Autodesk Fusion 360 part; units mm, degrees
(part 2 of 2)
  constraint symmetric L8 A252 A259
  constraint symmetric L8 L179.end A261.start
  constraint symmetric L8 L180.start L183.start
  constraint symmetric L8 A253 A261
  constraint symmetric L8 L177.end L184.end
  constraint symmetric L8 L178.start L182.start
  constraint symmetric L8 A254 A263
  constraint symmetric L8 L178.end L182.end
  constraint symmetric L8 L179.start L185.start
  constraint symmetric L8 A255 A262
  constraint symmetric L8 A256 A260
  constraint symmetric L8 A257 A258
  constraint symmetric L8 A264 A265
  constraint symmetric L7 A264 A267
  constraint symmetric L7 A265 A266
  measures "d1" diameter of A0
  measures "d2" distance of L0.start L0.end
  measures "d3" distance of L0.start L2.end
  measures "d4" diameter of A1
  measures "d5" diameter of A2
  measures "d6" diameter of A3
  measures "d7" distance of L1 A3.centre
  measures "d8" distance of L3 A2.centre
  measures "d9" distance of A0.centre L0
  measures "d10" distance of L2 A2.centre
  measures "d11" distance of L1 L4
  measures "d12" diameter of A4
  measures "d13" distance of A4.centre L6
  measures "d15" distance of L9.start L11.end L6.end
  measures "d16" distance of L1 L18
  measures "d17" distance of L15 L17
  measures "d18" distance of L19.start L19.end
  measures "d19" distance of L23.end L24.end
  measures "d20" distance of L23.start L23.end
  measures "d21" distance of L19 L21
  measures "d22" diameter of A5
  measures "d26" distance of L12 L26
  measures "d27" distance of L9 L27
  measures "d28" distance of L10 L12
  measures "d29" distance of L26 L41
  measures "d30" distance of L23 L40
  measures "d31" radius of A6
  measures "d32" radius of A8
  measures "d33" radius of A10
  measures "d34" distance of L68 L71
  measures "d35" radius of A33
  measures "d36" distance of A36.centre A35.centre
  measures "d37" radius of A35
  measures "d40" diameter of A47
  measures "d41" diameter of A48
  measures "d42" diameter of A49
  measures "d43" diameter of A50
  measures "d44" diameter of A51
  measures "d45" distance of A52.centre A51.centre
  measures "d46" distance of L73 A52.centre
  measures "d47" distance of L71 L81
  measures "d48" diameter of A53
  measures "d49" distance of L68 L84
  measures "d50" diameter of A59
  measures "d51" distance of L8 A59.centre
  measures "d56" distance of L68 A59.centre
  measures "d57" diameter of A60
  measures "d58" vertical distance of A59.centre A60.centre
  measures "d59" distance of L8 A60.centre
  measures "d60" diameter of A63
  measures "d61" diameter of A64
  measures "d62" angle of L89 L90
  measures "d63" distance of L7 A63.centre
  measures "d64" distance of L7 A64.centre
  measures "d65" diameter of A71
  measures "d66" diameter of A72
  measures "d67" distance of A73.centre A72.centre
  measures "d68" distance of L12 L93
  measures "d70" diameter of A74
  measures "d72" diameter of A75
  measures "d73" vertical distance of A73.centre A75.centre
  measures "d74" distance of A72.centre A74.centre
  measures "d75" diameter of A86
  measures "d76" distance of A87.centre A86.centre
  measures "d77" distance of L12 L102
  measures "d78" distance of L40 A86.centre
  measures "d79" diameter of A90
  measures "d80" distance of L45 L107
  measures "d81" distance of A91.centre A90.centre
  measures "d82" diameter of A92
  measures "d83" distance of A90.centre A92.centre L6.end
  measures "d84" diameter of A93
  measures "d85" distance of A94.centre A93.centre
  measures "d86" distance of A92.centre A94.centre
  measures "d87" diameter of A95
  measures "d88" distance of A93.centre A95.centre
  measures "d89" diameter of A96
  measures "d90" distance of A95.centre A97.centre
  measures "d91" distance of A97.centre A96.centre
  measures "d92" diameter of A98
  measures "d93" distance of A96.centre A98.centre
  measures "d94" diameter of A106
  measures "d95" distance of L53 A106.centre
  measures "d100" diameter of A107
  measures "d101" distance of L68 A107.centre
  measures "d102" diameter of A108
  measures "d103" diameter of A109
  measures "d104" distance of A108.centre A109.centre
  measures "d105" vertical distance of A5.centre A109.centre
  measures "d106" diameter of A111
  measures "d107" diameter of A110
  measures "d108" distance of A110.centre A111.centre
  measures "d109" vertical distance of A107.centre A111.centre
  measures "d110" diameter of A118
  measures "d111" diameter of A117
  measures "d112" distance of A118.centre A117.centre
  measures "d113" vertical distance of A31.centre A118.centre
  measures "d114" diameter of A121
  measures "d116" distance of L8 A121.centre
  measures "d117" vertical distance of A36.centre A121.centre
  measures "d118" diameter of A123
  measures "d119" diameter of A124
  measures "d120" angle of L119 L120
  measures "d121" diameter of A125
  measures "d122" diameter of A126
  measures "d123" diameter of A127
  measures "d124" diameter of A128
  measures "d127" distance of L45 A123.centre
  measures "d128" distance of P1 P2
  measures "d129" distance of P1 P3
  measures "d130" radius of A134
  measures "d131" diameter of A138
  measures "d132" distance of L121 A138.centre
  measures "d133" distance of L124 A138.centre
  measures "d134" diameter of A140
  measures "d135" distance of L121 A140.centre
  measures "d136" distance of A138.centre A140.centre
  measures "d137" angle of L127 L128
  measures "d138" distance of L127.start L127.end
  measures "d139" diameter of A154
  measures "d140" diameter of A155
  measures "d141" distance of A154.centre A155.centre
  measures "d142" distance of L121 A155.centre
  measures "d143" diameter of A156 L6.end
  measures "d144" diameter of A157
  measures "d145" distance of A156.centre A157.centre
  measures "d146" distance of L7 A157.centre
  measures "d149" diameter of A184
  measures "d150" distance of L9 A184.centre
  measures "d151" distance of L8 A184.centre
  measures "d152" diameter of A186
  measures "d153" distance of L72 A186.centre
  measures "d154" distance of L71 A186.centre
  measures "d155" diameter of A188
  measures "d156" distance of L47 A188.centre
  measures "d157" distance of L10 A188.centre
  measures "d158" diameter of A190
  measures "d159" distance of L66 A190.centre
  measures "d160" distance of L12 A190.centre
  measures "d163" diameter of A191
  measures "d164" distance of L42 A191.centre
  measures "d165" diameter of A201
  measures "d166" distance of L68 A201.centre
  measures "d169" distance of L143.start L143.end
  measures "d170" distance of L143.start L145.end
  measures "d171" diameter of A207
  measures "d172" distance of L147.start L147.end
  measures "d173" distance of L12 L144
  measures "d176" diameter of A216
  measures "d177" vertical distance of A157.centre P8
  measures "d179" diameter of A217
  measures "d180" angle of L157 L158
  measures "d181" diameter of A218
  measures "d182" angle of L159 L160
  measures "d183" diameter of A222
  measures "d184" radius of A227
  measures "d186" distance of A226.end L162.end
  measures "d187" distance of L7 L163
  measures "d188" diameter of A228
  measures "d189" distance of L12 A228.centre
  measures "d190" distance of L61 A228.centre
  measures "d191" diameter of A229
  measures "d192" distance of L12 A229.centre
  measures "d193" diameter of A230
  measures "d194" distance of A229.centre A230.centre
  measures "d195" diameter of A231
  measures "d196" distance of A228.centre A231.centre
  measures "d197" diameter of A232
  measures "d198" distance of A231.centre A232.centre
  measures "d199" diameter of A233
  measures "d200" distance of A231.centre A233.centre
  measures "d201" diameter of A234
  measures "d202" distance of A232.centre A234.centre
  measures "d203" diameter of A235
  measures "d204" diameter of A236
  measures "d205" diameter of A237
  measures "d206" distance of A232.centre A235.centre
  measures "d207" distance of A235.centre A237.centre
  measures "d208" diameter of A238
  measures "d209" distance of L164.start L164.end
  measures "d212" diameter of A242
  measures "d213" diameter of A243
  measures "d214" distance of A242.centre A243.centre
  measures "d215" distance of L8 A242.centre
  measures "d216" distance of L7 A242.centre
  measures "d221" diameter of A246
  measures "d222" distance of A246.end L170.end
  measures "d223" diameter of A248
  measures "d224" distance of L172.start L172.end
  measures "d225" distance of P10 P11
  measures "d226" distance of P10 P12
  measures "d227" radius of A252
  measures "d228" diameter of A256
  measures "d229" diameter of A257
  measures "d230" horizontal distance of A256.centre A257.centre
  measures "d231" diameter of A264
extrude "拉伸9" add sketch "草图1" along normal blind 3
sketch "草图5" plane through (0, 0, 3) normal (0, 0, 1) x (-1, 0, 0)
  circle A0 centre (-65.0738, -123.4519) radius 11
  circle A1 centre (-71.75, -44.17) radius 1.3
  circle A2 centre (24.5, 82.5) radius 1.6
  circle A3 centre (-112.5, 146) radius 1.6
  circle A4 centre (86, 58.5) radius 2.1
  circle A5 centre (-30.5, -30.5) radius 2.1
  circle A6 centre (-92.25, -44.17) radius 1.3
  arc A7 (74.1958, 45) -> (74.1958, 35) centre (74.1958, 40) ccw
  line L0 (74.1958, 45) -> (89.1958, 45)
  arc A8 (89.1958, 35) -> (89.1958, 45) centre (89.1958, 40) ccw
  line L1 (89.1958, 35) -> (74.1958, 35)
  arc A9 (-62, -15) -> (-58, -15) centre (-60, -15) ccw
  line L2 (-62, -15) -> (-62, 15)
  arc A10 (-58, 15) -> (-62, 15) centre (-60, 15) ccw
  line L3 (-58, 15) -> (-58, -15)
  circle A11 centre (-24.5, 62.5) radius 1.6
  circle A12 centre (-40, 140) radius 2.1
  arc A13 (7.5, 42) -> (7.5, 52) centre (7.5, 47) ccw
  line L4 (7.5, 42) -> (-7.5, 42)
  arc A14 (-7.5, 52) -> (-7.5, 42) centre (-7.5, 47) ccw
  line L5 (-7.5, 52) -> (7.5, 52)
  arc A15 (75, 147.55) -> (75, 144.45) centre (75, 146) ccw
  line L6 (75, 147.55) -> (105, 147.55)
  arc A16 (105, 144.45) -> (105, 147.55) centre (105, 146) ccw
  line L7 (105, 144.45) -> (75, 144.45)
  circle A17 centre (30.5, -30.5) radius 2.1
  circle A18 centre (39, 126) radius 1.6
  circle A19 centre (-35, -5) radius 1.5
  circle A20 centre (23.5589, -105.2416) radius 1.6
  circle A21 centre (23.5589, -124.7584) radius 1.6
  circle A22 centre (-9.7584, -91.4411) radius 1.6
  arc A23 (116.45, 131.5) -> (119.55, 131.5) centre (118, 131.5) ccw
  line L8 (116.45, 131.5) -> (116.45, 141.5)
  arc A24 (119.55, 141.5) -> (116.45, 141.5) centre (118, 141.5) ccw
  line L9 (119.55, 141.5) -> (119.55, 131.5)
  circle A25 centre (-112, -35.5) radius 2.1
  circle A26 centre (-24.5, 140.5) radius 1.6
  circle A27 centre (65.0738, -123.4519) radius 11
  circle A28 centre (115.49, -47.48) radius 1.6
  circle A29 centre (91, 86) radius 2.1
  circle A30 centre (-91, 86) radius 2.1
  circle A31 centre (-24.5, 120.5) radius 1.6
  circle A32 centre (112, -35.5) radius 2.1
  circle A33 centre (30.5, 30.5) radius 2.1
  line L10 (102, -15) -> (102, 15)
  arc A34 (106, 15) -> (102, 15) centre (104, 15) ccw
  line L11 (106, 15) -> (106, -15)
  arc A35 (102, -15) -> (106, -15) centre (104, -15) ccw
  circle A36 centre (86, -58.5) radius 2.1
  circle A37 centre (-40, -140) radius 2.1
  circle A38 centre (19, 77) radius 1.6
  circle A39 centre (-37.78, 121.07) radius 1.6
  circle A40 centre (37.78, 69) radius 1.6
  circle A41 centre (92.25, -44.17) radius 1.3
  arc A42 (-74.5, -40.2) -> (-74.7, -40) centre (-74.7, -40.2) ccw
  line L12 (-74.5, -40.2) -> (-74.5, -48.14)
  arc A43 (-74.7, -48.34) -> (-74.5, -48.14) centre (-74.7, -48.14) ccw
  line L13 (-74.7, -48.34) -> (-89.3, -48.34)
  arc A44 (-89.5, -48.14) -> (-89.3, -48.34) centre (-89.3, -48.14) ccw
  line L14 (-89.5, -48.14) -> (-89.5, -40.2)
  arc A45 (-89.3, -40) -> (-89.5, -40.2) centre (-89.3, -40.2) ccw
  line L15 (-89.3, -40) -> (-74.7, -40)
  circle A46 centre (24.5, 62.5) radius 1.6
  arc A47 (-106, -15) -> (-102, -15) centre (-104, -15) ccw
  line L16 (-106, -15) -> (-106, 15)
  arc A48 (-102, 15) -> (-106, 15) centre (-104, 15) ccw
  line L17 (-102, 15) -> (-102, -15)
  circle A49 centre (37.78, 121.07) radius 1.6
  circle A50 centre (-39, 126) radius 1.6
  circle A51 centre (-23.5589, -124.7584) radius 1.6
  circle A52 centre (-23.5589, -105.2416) radius 1.6
  circle A53 centre (24.5, 140.5) radius 1.6
  circle A54 centre (-65.0738, 123.4519) radius 11
  arc A55 (89.3, -48.34) -> (89.5, -48.14) centre (89.3, -48.14) ccw
  line L18 (89.3, -48.34) -> (74.7, -48.34)
  arc A56 (74.5, -48.14) -> (74.7, -48.34) centre (74.7, -48.14) ccw
  line L19 (74.5, -48.14) -> (74.5, -40.2)
  arc A57 (74.7, -40) -> (74.5, -40.2) centre (74.7, -40.2) ccw
  line L20 (74.7, -40) -> (89.3, -40)
  arc A58 (89.5, -40.2) -> (89.3, -40) centre (89.3, -40.2) ccw
  line L21 (89.5, -40.2) -> (89.5, -48.14)
  circle A59 centre (40, 140) radius 2.1
  circle A60 centre (-24.5, 82.5) radius 1.6
  circle A61 centre (112, 35.5) radius 2.1
  circle A62 centre (-5, 61.5) radius 1.5
  circle A63 centre (35, 5) radius 1.5
  circle A64 centre (9.7584, -91.4411) radius 1.6
  circle A65 centre (-37.78, 69) radius 1.6
  arc A66 (77, -7.5) -> (87, -7.5) centre (82, -7.5) ccw
  line L22 (77, -7.5) -> (77, 7.5)
  arc A67 (87, 7.5) -> (77, 7.5) centre (82, 7.5) ccw
  line L23 (87, 7.5) -> (87, -7.5)
  circle A68 centre (35, -5) radius 1.5
  circle A69 centre (19, 126) radius 1.6
  circle A70 centre (43.1, -93.2) radius 1.6
  circle A71 centre (5, -35) radius 1.5
  circle A72 centre (86, 113.5) radius 2.1
  circle A73 centre (-86, -58.5) radius 2.1
  circle A74 centre (43.1, -47.48) radius 1.6
  circle A75 centre (5, 35) radius 1.5
  arc A76 (-77, 7.5) -> (-87, 7.5) centre (-82, 7.5) ccw
  line L24 (-77, 7.5) -> (-77, -7.5)
  arc A77 (-87, -7.5) -> (-77, -7.5) centre (-82, -7.5) ccw
  line L25 (-87, -7.5) -> (-87, 7.5)
  circle A78 centre (67.5, 146) radius 1.6
  circle A79 centre (71.75, -44.17) radius 1.3
  circle A80 centre (-19, 77) radius 1.6
  arc A81 (7.5, -71) -> (7.5, -61) centre (7.5, -66) ccw
  line L26 (7.5, -71) -> (-7.5, -71)
  arc A82 (-7.5, -61) -> (-7.5, -71) centre (-7.5, -66) ccw
  line L27 (-7.5, -61) -> (7.5, -61)
  circle A83 centre (-30.5, 30.5) radius 2.1
  circle A84 centre (-5, 35) radius 1.5
  circle A85 centre (-35, 5) radius 1.5
  circle A86 centre (24.5, 120.5) radius 1.6
  circle A87 centre (-19, 126) radius 1.6
  circle A88 centre (22.5, 146) radius 1.6
  arc A89 (-89.1958, 45) -> (-89.1958, 35) centre (-89.1958, 40) ccw
  line L28 (-89.1958, 45) -> (-74.1958, 45)
  arc A90 (-74.1958, 35) -> (-74.1958, 45) centre (-74.1958, 40) ccw
  line L29 (-74.1958, 35) -> (-89.1958, 35)
  circle A91 centre (112.5, 146) radius 1.6
  arc A92 (58, -15) -> (62, -15) centre (60, -15) ccw
  line L30 (58, -15) -> (58, 15)
  arc A93 (62, 15) -> (58, 15) centre (60, 15) ccw
  line L31 (62, 15) -> (62, -15)
  circle A94 centre (43.1, -113.52) radius 1.6
  circle A95 centre (40, -140) radius 2.1
  circle A96 centre (-9.7584, -138.5589) radius 1.6
  circle A97 centre (86, -113.5) radius 2.1
  circle A98 centre (91, -86) radius 2.1
  circle A99 centre (-22.5, 146) radius 1.6
  circle A100 centre (43.1, 110) radius 1.6
  circle A101 centre (39, 77) radius 1.6
  circle A102 centre (-5, -35) radius 1.5
  circle A103 centre (-39, 77) radius 1.6
  circle A104 centre (-86, 113.5) radius 2.1
  circle A105 centre (-86, 58.5) radius 2.1
  arc A106 (-75, 144.45) -> (-75, 147.55) centre (-75, 146) ccw
  line L32 (-75, 144.45) -> (-105, 144.45)
  arc A107 (-105, 147.55) -> (-105, 144.45) centre (-105, 146) ccw
  line L33 (-105, 147.55) -> (-75, 147.55)
  circle A108 centre (-86, -113.5) radius 2.1
  circle A109 centre (65.0738, 123.4519) radius 11
  circle A110 centre (9.7584, -138.5589) radius 1.6
  arc A111 (-30, 144.45) -> (-30, 147.55) centre (-30, 146) ccw
  line L34 (-30, 144.45) -> (-60, 144.45)
  arc A112 (-60, 147.55) -> (-60, 144.45) centre (-60, 146) ccw
  line L35 (-60, 147.55) -> (-30, 147.55)
  circle A113 centre (5, 61.5) radius 1.5
  arc A114 (30, 147.55) -> (30, 144.45) centre (30, 146) ccw
  line L36 (30, 147.55) -> (60, 147.55)
  arc A115 (60, 144.45) -> (60, 147.55) centre (60, 146) ccw
  line L37 (60, 144.45) -> (30, 144.45)
  circle A116 centre (-111.84, -47.48) radius 1.6
  arc A117 (-116.45, 141.5) -> (-119.55, 141.5) centre (-118, 141.5) ccw
  line L38 (-116.45, 141.5) -> (-116.45, 131.5)
  arc A118 (-119.55, 131.5) -> (-116.45, 131.5) centre (-118, 131.5) ccw
  line L39 (-119.55, 131.5) -> (-119.55, 141.5)
  circle A119 centre (-112, 35.5) radius 2.1
  arc A120 (15, 144.45) -> (15, 147.55) centre (15, 146) ccw
  line L40 (15, 144.45) -> (-15, 144.45)
  arc A121 (-15, 147.55) -> (-15, 144.45) centre (-15, 146) ccw
  line L41 (-15, 147.55) -> (15, 147.55)
  circle A122 centre (115.49, 110) radius 1.6
  circle A123 centre (-91, -86) radius 2.1
  circle A124 centre (-88.98, 110) radius 1.6
  circle A125 centre (-67.5, 146) radius 1.6
  circle A126 centre (-111.84, -93.2) radius 1.6
  circle A127 centre (22.5, 22.5) radius 1.55
  arc A128 (-30, -147.55) -> (-30, -144.45) centre (-30, -146) ccw
  line L42 (-30, -147.55) -> (-60, -147.55)
  arc A129 (-60, -144.45) -> (-60, -147.55) centre (-60, -146) ccw
  line L43 (-60, -144.45) -> (-30, -144.45)
  circle A130 centre (53, -101) radius 2.1
  circle A131 centre (45.5, 52.5) radius 1.5
  circle A132 centre (-6, -76.5) radius 1.5
  arc A133 (75, -144.45) -> (75, -147.55) centre (75, -146) ccw
  line L44 (75, -144.45) -> (105, -144.45)
  arc A134 (105, -147.55) -> (105, -144.45) centre (105, -146) ccw
  line L45 (105, -147.55) -> (75, -147.55)
  circle A135 centre (53, 101) radius 2.1
  circle A136 centre (-112, 140) radius 2.1
  circle A137 centre (78, 71) radius 2.1
  circle A138 centre (-14.0007, -129.0007) radius 1.3
  circle A139 centre (-35.5, 52.5) radius 1.5
  circle A140 centre (-78, -101) radius 2.1
  circle A141 centre (-53, 71) radius 2.1
  arc A142 (60, -147.55) -> (60, -144.45) centre (60, -146) ccw
  line L46 (60, -147.55) -> (30, -147.55)
  arc A143 (30, -144.45) -> (30, -147.55) centre (30, -146) ccw
  line L47 (30, -144.45) -> (60, -144.45)
  circle A144 centre (78, -101) radius 2.1
  circle A145 centre (-22.5, -146) radius 1.6
  circle A146 centre (-20.8597, -135.8596) radius 1.6
  circle A147 centre (-14.0007, -100.9993) radius 1.3
  circle A148 centre (53, 71) radius 2.1
  circle A149 centre (15.25, 15.25) radius 1.55
  circle A150 centre (22.5, -22.5) radius 1.55
  circle A151 centre (22.5, -146) radius 1.6
  arc A152 (8, 81) -> (8, 91) centre (8, 86) ccw
  line L48 (8, 81) -> (-8, 81)
  arc A153 (-8, 91) -> (-8, 81) centre (-8, 86) ccw
  line L49 (-8, 91) -> (8, 91)
  circle A154 centre (35.5, 52.5) radius 1.5
  circle A155 centre (14.0007, -129.0007) radius 1.3
  arc A156 (15, -147.55) -> (15, -144.45) centre (15, -146) ccw
  line L50 (15, -147.55) -> (-15, -147.55)
  arc A157 (-15, -144.45) -> (-15, -147.55) centre (-15, -146) ccw
  line L51 (-15, -144.45) -> (15, -144.45)
  circle A158 centre (112.5, -146) radius 1.6
  circle A159 centre (15.25, -15.25) radius 1.55
  circle A160 centre (-118, 0) radius 1.6
  circle A161 centre (-53, -101) radius 2.1
  circle A162 centre (-78, 101) radius 2.1
  arc A163 (-119.55, -141.5) -> (-116.45, -141.5) centre (-118, -141.5) ccw
  line L52 (-119.55, -141.5) -> (-119.55, -131.5)
  arc A164 (-116.45, -131.5) -> (-119.55, -131.5) centre (-118, -131.5) ccw
  line L53 (-116.45, -131.5) -> (-116.45, -141.5)
  arc A165 (-116.45, 32.5) -> (-119.55, 32.5) centre (-118, 32.5) ccw
  line L54 (-116.45, 32.5) -> (-116.45, 7.5)
  arc A166 (-119.55, 7.5) -> (-116.45, 7.5) centre (-118, 7.5) ccw
  line L55 (-119.55, 7.5) -> (-119.55, 32.5)
  circle A167 centre (118, 40) radius 1.6
  arc A168 (116.45, -141.5) -> (119.55, -141.5) centre (118, -141.5) ccw
  line L56 (116.45, -141.5) -> (116.45, -131.5)
  arc A169 (119.55, -131.5) -> (116.45, -131.5) centre (118, -131.5) ccw
  line L57 (119.55, -131.5) -> (119.55, -141.5)
  circle A170 centre (118, -40) radius 1.6
  circle A171 centre (78, 101) radius 2.1
  circle A172 centre (67.5, -146) radius 1.6
  circle A173 centre (0, -135) radius 5
  circle A174 centre (-40.5, 61) radius 5
  circle A175 centre (112, -140) radius 2.1
  circle A176 centre (-20.8597, -94.1403) radius 1.6
  arc A177 (-75, -147.55) -> (-75, -144.45) centre (-75, -146) ccw
  line L58 (-75, -147.55) -> (-105, -147.55)
  arc A178 (-105, -144.45) -> (-105, -147.55) centre (-105, -146) ccw
  line L59 (-105, -144.45) -> (-75, -144.45)
  circle A179 centre (78, -71) radius 2.1
  circle A180 centre (-112, -140) radius 2.1
  circle A181 centre (20.8596, -135.8597) radius 1.6
  circle A182 centre (-53, -71) radius 2.1
  circle A183 centre (-78, -71) radius 2.1
  circle A184 centre (-118, 40) radius 1.6
  circle A185 centre (-22.5, 22.5) radius 1.55
  circle A186 centre (14.0007, -100.9993) radius 1.3
  arc A187 (119.55, -7.5) -> (116.45, -7.5) centre (118, -7.5) ccw
  line L60 (119.55, -7.5) -> (119.55, -32.5)
  arc A188 (116.45, -32.5) -> (119.55, -32.5) centre (118, -32.5) ccw
  line L61 (116.45, -32.5) -> (116.45, -7.5)
  circle A189 centre (40.5, 61) radius 5
  arc A190 (-119.55, -32.5) -> (-116.45, -32.5) centre (-118, -32.5) ccw
  line L62 (-119.55, -32.5) -> (-119.55, -7.5)
  arc A191 (-116.45, -7.5) -> (-119.55, -7.5) centre (-118, -7.5) ccw
  line L63 (-116.45, -7.5) -> (-116.45, -32.5)
  circle A192 centre (-53, 101) radius 2.1
  circle A193 centre (-112.5, -146) radius 1.6
  circle A194 centre (-78, 71) radius 2.1
  circle A195 centre (-22.5, -22.5) radius 1.55
  circle A196 centre (-15.25, 15.25) radius 1.55
  circle A197 centre (-118, -40) radius 1.6
  circle A198 centre (53, -71) radius 2.1
  circle A199 centre (118, 0) radius 1.6
  circle A200 centre (-15.25, -15.25) radius 1.55
  circle A201 centre (20.8596, -94.1403) radius 1.6
  circle A202 centre (0, 0) radius 5
  circle A203 centre (-45.5, 52.5) radius 1.5
  arc A204 (116.45, 7.5) -> (119.55, 7.5) centre (118, 7.5) ccw
  line L64 (116.45, 7.5) -> (116.45, 32.5)
  arc A205 (119.55, 32.5) -> (116.45, 32.5) centre (118, 32.5) ccw
  line L65 (119.55, 32.5) -> (119.55, 7.5)
  circle A206 centre (-67.5, -146) radius 1.6
  circle A207 centre (6, -76.5) radius 1.5
  circle A208 centre (112, 140) radius 2.1
  line L66 (-122, 140) -> (-122, -140)
  arc A209 (-122, -140) -> (-112, -150) centre (-112, -140) ccw
  line L67 (-112, -150) -> (0, -150)
  line L68 (0, -150) -> (112, -150)
  arc A210 (112, -150) -> (122, -140) centre (112, -140) ccw
  line L69 (122, -140) -> (122, -131.5)
  line L70 (122, -131.5) -> (122, -40.5)
  line L71 (122, -40.5) -> (122, 0)
  line L72 (122, 0) -> (122, 40.5)
  line L73 (122, 40.5) -> (122, 131.5)
  line L74 (122, 131.5) -> (122, 140)
  arc A211 (122, 140) -> (112, 150) centre (112, 140) ccw
  line L75 (112, 150) -> (0, 150)
  line L76 (0, 150) -> (-112, 150)
  arc A212 (-112, 150) -> (-122, 140) centre (-112, 140) ccw
  line L77 (0, 0) -> (0, -164.8837) construction
  circle A213 centre (-18, -129.0007) radius 1.6
  circle A214 centre (18, -129.0007) radius 1.6
  circle A215 centre (-18, -81.0007) radius 1.6
  circle A216 centre (18, -81.0007) radius 1.6
  dimension "d234" = 3.2
  dimension "d235" = 3.2
  dimension "d236" = 36
  dimension "d237" = 48
  constraint coincident A202.centre L77.start
  constraint perpendicular L27 L77
  constraint symmetric L77 A213 A214
  constraint vertical A213.centre A215.centre
  constraint symmetric L77 A215 A216
  constraint horizontal A138.centre A213.centre
  measures "d234" diameter of A213
  measures "d235" diameter of A215
  measures "d236" distance of A213.centre A214.centre
  measures "d237" distance of A213.centre A215.centre
extrude "拉伸10" cut sketch "草图5" against normal blind 3 contours A213 | A214 | A215 | A216
sketch "草图7" plane through (0, 0, 0) normal (0, 0, 1) x (1, 0, 0)
  circle A0 centre (-18, 129.0007) radius 1.6
  circle A1 centre (-18, 81.0007) radius 1.6
  circle A2 centre (18, 129.0007) radius 1.6
  circle A3 centre (18, 81.0007) radius 1.6
  circle A4 centre (65.0738, 123.4519) radius 11
  circle A5 centre (71.75, 44.17) radius 1.3
  circle A6 centre (-24.5, -82.5) radius 1.6
  circle A7 centre (112.5, -146) radius 1.6
  circle A8 centre (-86, -58.5) radius 2.1
  circle A9 centre (30.5, 30.5) radius 2.1
  circle A10 centre (92.25, 44.17) radius 1.3
  arc A11 (-74.1958, -45) -> (-74.1958, -35) centre (-74.1958, -40) ccw
  line L0 (-74.1958, -45) -> (-89.1958, -45)
  arc A12 (-89.1958, -35) -> (-89.1958, -45) centre (-89.1958, -40) ccw
  line L1 (-89.1958, -35) -> (-74.1958, -35)
  arc A13 (62, 15) -> (58, 15) centre (60, 15) ccw
  line L2 (62, 15) -> (62, -15)
  arc A14 (58, -15) -> (62, -15) centre (60, -15) ccw
  line L3 (58, -15) -> (58, 15)
  circle A15 centre (24.5, -62.5) radius 1.6
  circle A16 centre (40, -140) radius 2.1
  arc A17 (-7.5, -42) -> (-7.5, -52) centre (-7.5, -47) ccw
  line L4 (-7.5, -42) -> (7.5, -42)
  arc A18 (7.5, -52) -> (7.5, -42) centre (7.5, -47) ccw
  line L5 (7.5, -52) -> (-7.5, -52)
  arc A19 (-75, -147.55) -> (-75, -144.45) centre (-75, -146) ccw
  line L6 (-75, -147.55) -> (-105, -147.55)
  arc A20 (-105, -144.45) -> (-105, -147.55) centre (-105, -146) ccw
  line L7 (-105, -144.45) -> (-75, -144.45)
  circle A21 centre (-30.5, 30.5) radius 2.1
  circle A22 centre (-39, -126) radius 1.6
  circle A23 centre (35, 5) radius 1.5
  circle A24 centre (-23.5589, 105.2416) radius 1.6
  circle A25 centre (-23.5589, 124.7584) radius 1.6
  circle A26 centre (9.7584, 91.4411) radius 1.6
  arc A27 (-116.45, -131.5) -> (-119.55, -131.5) centre (-118, -131.5) ccw
  line L8 (-116.45, -131.5) -> (-116.45, -141.5)
  arc A28 (-119.55, -141.5) -> (-116.45, -141.5) centre (-118, -141.5) ccw
  line L9 (-119.55, -141.5) -> (-119.55, -131.5)
  circle A29 centre (112, 35.5) radius 2.1
  circle A30 centre (24.5, -140.5) radius 1.6
  circle A31 centre (-65.0738, 123.4519) radius 11
  circle A32 centre (-115.49, 47.48) radius 1.6
  circle A33 centre (-91, -86) radius 2.1
  circle A34 centre (91, -86) radius 2.1
  circle A35 centre (24.5, -120.5) radius 1.6
  circle A36 centre (-112, 35.5) radius 2.1
  circle A37 centre (-30.5, -30.5) radius 2.1
  line L10 (-102, 15) -> (-102, -15)
  arc A38 (-106, -15) -> (-102, -15) centre (-104, -15) ccw
  line L11 (-106, -15) -> (-106, 15)
  arc A39 (-102, 15) -> (-106, 15) centre (-104, 15) ccw
  circle A40 centre (-86, 58.5) radius 2.1
  circle A41 centre (40, 140) radius 2.1
  circle A42 centre (-19, -77) radius 1.6
  circle A43 centre (37.78, -121.07) radius 1.6
  circle A44 centre (-37.78, -69) radius 1.6
  circle A45 centre (-92.25, 44.17) radius 1.3
  arc A46 (74.5, 40.2) -> (74.7, 40) centre (74.7, 40.2) ccw
  line L12 (74.5, 40.2) -> (74.5, 48.14)
  arc A47 (74.7, 48.34) -> (74.5, 48.14) centre (74.7, 48.14) ccw
  line L13 (74.7, 48.34) -> (89.3, 48.34)
  arc A48 (89.5, 48.14) -> (89.3, 48.34) centre (89.3, 48.14) ccw
  line L14 (89.5, 48.14) -> (89.5, 40.2)
  arc A49 (89.3, 40) -> (89.5, 40.2) centre (89.3, 40.2) ccw
  line L15 (89.3, 40) -> (74.7, 40)
  circle A50 centre (-24.5, -62.5) radius 1.6
  arc A51 (106, 15) -> (102, 15) centre (104, 15) ccw
  line L16 (106, 15) -> (106, -15)
  arc A52 (102, -15) -> (106, -15) centre (104, -15) ccw
  line L17 (102, -15) -> (102, 15)
  circle A53 centre (-37.78, -121.07) radius 1.6
  circle A54 centre (39, -126) radius 1.6
  circle A55 centre (23.5589, 124.7584) radius 1.6
  circle A56 centre (23.5589, 105.2416) radius 1.6
  circle A57 centre (-24.5, -140.5) radius 1.6
  circle A58 centre (65.0738, -123.4519) radius 11
  arc A59 (-89.3, 48.34) -> (-89.5, 48.14) centre (-89.3, 48.14) ccw
  line L18 (-89.3, 48.34) -> (-74.7, 48.34)
  arc A60 (-74.5, 48.14) -> (-74.7, 48.34) centre (-74.7, 48.14) ccw
  line L19 (-74.5, 48.14) -> (-74.5, 40.2)
  arc A61 (-74.7, 40) -> (-74.5, 40.2) centre (-74.7, 40.2) ccw
  line L20 (-74.7, 40) -> (-89.3, 40)
  arc A62 (-89.5, 40.2) -> (-89.3, 40) centre (-89.3, 40.2) ccw
  line L21 (-89.5, 40.2) -> (-89.5, 48.14)
  circle A63 centre (-40, -140) radius 2.1
  circle A64 centre (24.5, -82.5) radius 1.6
  circle A65 centre (-112, -35.5) radius 2.1
  circle A66 centre (5, -61.5) radius 1.5
  circle A67 centre (-35, -5) radius 1.5
  circle A68 centre (-9.7584, 91.4411) radius 1.6
  circle A69 centre (37.78, -69) radius 1.6
  arc A70 (-77, 7.5) -> (-87, 7.5) centre (-82, 7.5) ccw
  line L22 (-77, 7.5) -> (-77, -7.5)
  arc A71 (-87, -7.5) -> (-77, -7.5) centre (-82, -7.5) ccw
  line L23 (-87, -7.5) -> (-87, 7.5)
  circle A72 centre (-35, 5) radius 1.5
  circle A73 centre (-19, -126) radius 1.6
  circle A74 centre (-43.1, 93.2) radius 1.6
  circle A75 centre (-5, 35) radius 1.5
  circle A76 centre (-86, -113.5) radius 2.1
  circle A77 centre (86, 58.5) radius 2.1
  circle A78 centre (-43.1, 47.48) radius 1.6
  circle A79 centre (-5, -35) radius 1.5
  arc A80 (77, -7.5) -> (87, -7.5) centre (82, -7.5) ccw
  line L24 (77, -7.5) -> (77, 7.5)
  arc A81 (87, 7.5) -> (77, 7.5) centre (82, 7.5) ccw
  line L25 (87, 7.5) -> (87, -7.5)
  circle A82 centre (-67.5, -146) radius 1.6
  circle A83 centre (-71.75, 44.17) radius 1.3
  circle A84 centre (19, -77) radius 1.6
  arc A85 (-7.5, 71) -> (-7.5, 61) centre (-7.5, 66) ccw
  line L26 (-7.5, 71) -> (7.5, 71)
  arc A86 (7.5, 61) -> (7.5, 71) centre (7.5, 66) ccw
  line L27 (7.5, 61) -> (-7.5, 61)
  circle A87 centre (30.5, -30.5) radius 2.1
  circle A88 centre (5, -35) radius 1.5
  circle A89 centre (35, -5) radius 1.5
  circle A90 centre (-24.5, -120.5) radius 1.6
  circle A91 centre (19, -126) radius 1.6
  circle A92 centre (-22.5, -146) radius 1.6
  arc A93 (89.1958, -45) -> (89.1958, -35) centre (89.1958, -40) ccw
  line L28 (89.1958, -45) -> (74.1958, -45)
  arc A94 (74.1958, -35) -> (74.1958, -45) centre (74.1958, -40) ccw
  line L29 (74.1958, -35) -> (89.1958, -35)
  circle A95 centre (-112.5, -146) radius 1.6
  arc A96 (-58, 15) -> (-62, 15) centre (-60, 15) ccw
  line L30 (-58, 15) -> (-58, -15)
  arc A97 (-62, -15) -> (-58, -15) centre (-60, -15) ccw
  line L31 (-62, -15) -> (-62, 15)
  circle A98 centre (-43.1, 113.52) radius 1.6
  circle A99 centre (-40, 140) radius 2.1
  circle A100 centre (9.7584, 138.5589) radius 1.6
  circle A101 centre (-86, 113.5) radius 2.1
  circle A102 centre (-91, 86) radius 2.1
  circle A103 centre (22.5, -146) radius 1.6
  circle A104 centre (-43.1, -110) radius 1.6
  circle A105 centre (-39, -77) radius 1.6
  circle A106 centre (5, 35) radius 1.5
  circle A107 centre (39, -77) radius 1.6
  circle A108 centre (86, -113.5) radius 2.1
  circle A109 centre (86, -58.5) radius 2.1
  arc A110 (75, -144.45) -> (75, -147.55) centre (75, -146) ccw
  line L32 (75, -144.45) -> (105, -144.45)
  arc A111 (105, -147.55) -> (105, -144.45) centre (105, -146) ccw
  line L33 (105, -147.55) -> (75, -147.55)
  circle A112 centre (86, 113.5) radius 2.1
  circle A113 centre (-65.0738, -123.4519) radius 11
  circle A114 centre (-9.7584, 138.5589) radius 1.6
  arc A115 (30, -144.45) -> (30, -147.55) centre (30, -146) ccw
  line L34 (30, -144.45) -> (60, -144.45)
  arc A116 (60, -147.55) -> (60, -144.45) centre (60, -146) ccw
  line L35 (60, -147.55) -> (30, -147.55)
  circle A117 centre (-5, -61.5) radius 1.5
  arc A118 (-30, -147.55) -> (-30, -144.45) centre (-30, -146) ccw
  line L36 (-30, -147.55) -> (-60, -147.55)
  arc A119 (-60, -144.45) -> (-60, -147.55) centre (-60, -146) ccw
  line L37 (-60, -144.45) -> (-30, -144.45)
  circle A120 centre (111.84, 47.48) radius 1.6
  arc A121 (116.45, -141.5) -> (119.55, -141.5) centre (118, -141.5) ccw
  line L38 (116.45, -141.5) -> (116.45, -131.5)
  arc A122 (119.55, -131.5) -> (116.45, -131.5) centre (118, -131.5) ccw
  line L39 (119.55, -131.5) -> (119.55, -141.5)
  circle A123 centre (112, -35.5) radius 2.1
  arc A124 (-15, -144.45) -> (-15, -147.55) centre (-15, -146) ccw
  line L40 (-15, -144.45) -> (15, -144.45)
  arc A125 (15, -147.55) -> (15, -144.45) centre (15, -146) ccw
  line L41 (15, -147.55) -> (-15, -147.55)
  circle A126 centre (-115.49, -110) radius 1.6
  circle A127 centre (91, 86) radius 2.1
  circle A128 centre (88.98, -110) radius 1.6
  circle A129 centre (67.5, -146) radius 1.6
  circle A130 centre (111.84, 93.2) radius 1.6
  circle A131 centre (-22.5, -22.5) radius 1.55
  arc A132 (30, 147.55) -> (30, 144.45) centre (30, 146) ccw
  line L42 (30, 147.55) -> (60, 147.55)
  arc A133 (60, 144.45) -> (60, 147.55) centre (60, 146) ccw
  line L43 (60, 144.45) -> (30, 144.45)
  circle A134 centre (-53, 101) radius 2.1
  circle A135 centre (-45.5, -52.5) radius 1.5
  circle A136 centre (6, 76.5) radius 1.5
  arc A137 (-75, 144.45) -> (-75, 147.55) centre (-75, 146) ccw
  line L44 (-75, 144.45) -> (-105, 144.45)
  arc A138 (-105, 147.55) -> (-105, 144.45) centre (-105, 146) ccw
  line L45 (-105, 147.55) -> (-75, 147.55)
  circle A139 centre (-53, -101) radius 2.1
  circle A140 centre (112, -140) radius 2.1
  circle A141 centre (-78, -71) radius 2.1
  circle A142 centre (14.0007, 129.0007) radius 1.3
  circle A143 centre (35.5, -52.5) radius 1.5
  circle A144 centre (78, 101) radius 2.1
  circle A145 centre (53, -71) radius 2.1
  arc A146 (-60, 147.55) -> (-60, 144.45) centre (-60, 146) ccw
  line L46 (-60, 147.55) -> (-30, 147.55)
  arc A147 (-30, 144.45) -> (-30, 147.55) centre (-30, 146) ccw
  line L47 (-30, 144.45) -> (-60, 144.45)
  circle A148 centre (-78, 101) radius 2.1
  circle A149 centre (22.5, 146) radius 1.6
  circle A150 centre (20.8597, 135.8596) radius 1.6
  circle A151 centre (14.0007, 100.9993) radius 1.3
  circle A152 centre (-53, -71) radius 2.1
  circle A153 centre (-15.25, -15.25) radius 1.55
  circle A154 centre (-22.5, 22.5) radius 1.55
  circle A155 centre (-22.5, 146) radius 1.6
  arc A156 (-8, -81) -> (-8, -91) centre (-8, -86) ccw
  line L48 (-8, -81) -> (8, -81)
  arc A157 (8, -91) -> (8, -81) centre (8, -86) ccw
  line L49 (8, -91) -> (-8, -91)
  circle A158 centre (-35.5, -52.5) radius 1.5
  circle A159 centre (-14.0007, 129.0007) radius 1.3
  arc A160 (-15, 147.55) -> (-15, 144.45) centre (-15, 146) ccw
  line L50 (-15, 147.55) -> (15, 147.55)
  arc A161 (15, 144.45) -> (15, 147.55) centre (15, 146) ccw
  line L51 (15, 144.45) -> (-15, 144.45)
  circle A162 centre (-112.5, 146) radius 1.6
  circle A163 centre (-15.25, 15.25) radius 1.55
  circle A164 centre (118, 0) radius 1.6
  circle A165 centre (53, 101) radius 2.1
  circle A166 centre (78, -101) radius 2.1
  arc A167 (119.55, 141.5) -> (116.45, 141.5) centre (118, 141.5) ccw
  line L52 (119.55, 141.5) -> (119.55, 131.5)
  arc A168 (116.45, 131.5) -> (119.55, 131.5) centre (118, 131.5) ccw
  line L53 (116.45, 131.5) -> (116.45, 141.5)
  arc A169 (116.45, -32.5) -> (119.55, -32.5) centre (118, -32.5) ccw
  line L54 (116.45, -32.5) -> (116.45, -7.5)
  arc A170 (119.55, -7.5) -> (116.45, -7.5) centre (118, -7.5) ccw
  line L55 (119.55, -7.5) -> (119.55, -32.5)
  circle A171 centre (-118, -40) radius 1.6
  arc A172 (-116.45, 141.5) -> (-119.55, 141.5) centre (-118, 141.5) ccw
  line L56 (-116.45, 141.5) -> (-116.45, 131.5)
  arc A173 (-119.55, 131.5) -> (-116.45, 131.5) centre (-118, 131.5) ccw
  line L57 (-119.55, 131.5) -> (-119.55, 141.5)
  circle A174 centre (-118, 40) radius 1.6
  circle A175 centre (-78, -101) radius 2.1
  circle A176 centre (-67.5, 146) radius 1.6
  circle A177 centre (0, 135) radius 5
  circle A178 centre (40.5, -61) radius 5
  circle A179 centre (-112, 140) radius 2.1
  circle A180 centre (20.8597, 94.1403) radius 1.6
  arc A181 (75, 147.55) -> (75, 144.45) centre (75, 146) ccw
  line L58 (75, 147.55) -> (105, 147.55)
  arc A182 (105, 144.45) -> (105, 147.55) centre (105, 146) ccw
  line L59 (105, 144.45) -> (75, 144.45)
  circle A183 centre (-78, 71) radius 2.1
  circle A184 centre (112, 140) radius 2.1
  circle A185 centre (-20.8596, 135.8597) radius 1.6
  circle A186 centre (53, 71) radius 2.1
  circle A187 centre (78, 71) radius 2.1
  circle A188 centre (118, -40) radius 1.6
  circle A189 centre (22.5, -22.5) radius 1.55
  circle A190 centre (-14.0007, 100.9993) radius 1.3
  arc A191 (-119.55, 7.5) -> (-116.45, 7.5) centre (-118, 7.5) ccw
  line L60 (-119.55, 7.5) -> (-119.55, 32.5)
  arc A192 (-116.45, 32.5) -> (-119.55, 32.5) centre (-118, 32.5) ccw
  line L61 (-116.45, 32.5) -> (-116.45, 7.5)
  circle A193 centre (-40.5, -61) radius 5
  arc A194 (119.55, 32.5) -> (116.45, 32.5) centre (118, 32.5) ccw
  line L62 (119.55, 32.5) -> (119.55, 7.5)
  arc A195 (116.45, 7.5) -> (119.55, 7.5) centre (118, 7.5) ccw
  line L63 (116.45, 7.5) -> (116.45, 32.5)
  circle A196 centre (53, -101) radius 2.1
  circle A197 centre (112.5, 146) radius 1.6
  circle A198 centre (78, -71) radius 2.1
  circle A199 centre (22.5, 22.5) radius 1.55
  circle A200 centre (15.25, -15.25) radius 1.55
  circle A201 centre (118, 40) radius 1.6
  circle A202 centre (-53, 71) radius 2.1
  circle A203 centre (-118, 0) radius 1.6
  circle A204 centre (15.25, 15.25) radius 1.55
  circle A205 centre (-20.8596, 94.1403) radius 1.6
  circle A206 centre (0, 0) radius 5
  circle A207 centre (45.5, -52.5) radius 1.5
  arc A208 (-116.45, -7.5) -> (-119.55, -7.5) centre (-118, -7.5) ccw
  line L64 (-116.45, -7.5) -> (-116.45, -32.5)
  arc A209 (-119.55, -32.5) -> (-116.45, -32.5) centre (-118, -32.5) ccw
  line L65 (-119.55, -32.5) -> (-119.55, -7.5)
  circle A210 centre (67.5, 146) radius 1.6
  circle A211 centre (-6, 76.5) radius 1.5
  circle A212 centre (-112, -140) radius 2.1
  line L66 (122, -140) -> (122, 140)
  arc A213 (122, 140) -> (112, 150) centre (112, 140) ccw
  line L67 (112, 150) -> (0, 150)
  line L68 (0, 150) -> (-112, 150)
  arc A214 (-112, 150) -> (-122, 140) centre (-112, 140) ccw
  line L69 (-122, 140) -> (-122, 131.5)
  line L70 (-122, 131.5) -> (-122, 40.5)
  line L71 (-122, 40.5) -> (-122, 0)
  line L72 (-122, 0) -> (-122, -40.5)
  line L73 (-122, -40.5) -> (-122, -131.5)
  line L74 (-122, -131.5) -> (-122, -140)
  arc A215 (-122, -140) -> (-112, -150) centre (-112, -140) ccw
  line L75 (-112, -150) -> (0, -150)
  line L76 (0, -150) -> (112, -150)
  arc A216 (112, -150) -> (122, -140) centre (112, -140) ccw
equation "d26 = ( 32 / 2 ) * 1 mm"
equation "d51 = ( 41 / 2 ) * 1 mm"
equation "d57 = 5.5 mm + 0.3 mm"
equation "d59 = ( 32 / 2 ) * 1 mm"
equation "d63 = ( 30.5 / 2 ) * 1 mm"
equation "d64 = ( 45 / 2 ) * 1 mm"
equation "d116 = ( 12 / 2 ) * 1 mm"
equation "d180 = 90 deg - 22.5 deg"
equation "d189 = 10.16 mm + 22.86 mm"
equation "d192 = 10.16 mm + 154.94 mm"
equation "d198 = 154.94 mm - 22.86 mm"
equation "d215 = ( 75.56 / 2 ) * 1 mm"
equation "d226 = 8.1 mm + 0.24 mm"
